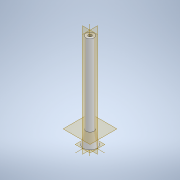
# Autodesk Inventor part: Towers
Saved by Autodesk Inventor 2022 (Build 260153000, 153)
## iProperties
Created: 2022-05-12
Part Number: Towers
Material: Generic
Document SubType Name: Modeling
Designer: dovalle
Density: 1 g/cm^3
Appearance: Default
Author: dovalle
Autodesk Inventor part; units mm, degrees
ref_plane "Work Plane1" through (0, 10, 0) normal (0, 1, 0) x (-1, 0, 0)
sketch "Sketch1" plane through (0, 0, 0) normal (0, 1, 0) x (-1, 0, 0)
  circle A0 centre (0, 0) radius 5
  constraints: 1 centre point, 1 coincident
sketch "Sketch2" plane through (0, 10, 0) normal (0, 1, 0) x (-1, 0, 0)
  circle A0 centre (0, 0) radius 3
  constraints: 1 centre point, 1 coincident
loft "Loft1" add profiles "Sketch2", "Sketch1"
sketch "Sketch3" plane through (0, 10, 0) normal (0, 1, 0) x (1, 0, 0)
  circle A0 centre (0, 0) radius 3
  constraints: 1 centre point, 1 coincident
extrude "Extrusion1" add sketch "Sketch3" along normal blind 60
sketch "Sketch4" plane through (0, 70, 0) normal (0, 1, 0) x (1, 0, 0)
  circle A0 centre (0, 0) radius 1.25
  constraints: 1 centre point, 1 coincident
extrude "Extrusion2" cut sketch "Sketch4" against normal blind 70
body "Solid1"
